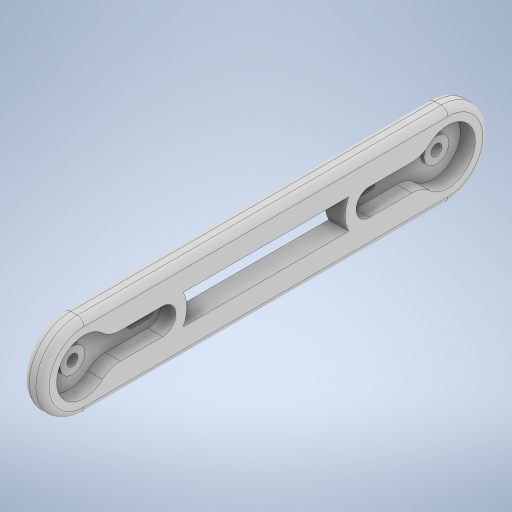
# Autodesk Inventor part: FemurHornSide
Saved by Autodesk Inventor 2024 (Build 280153000, 153)
## iProperties
Created: 2026-01-07
Part Number: FemurHornSide
Material: Generic
Document SubType Name: Modeling
Designer: Liam
Density: 1 g/cm^3
Appearance: Default
Mass: 22.8952 g
Surface Area: 100.934 cm^2
Volume: 22.8952 cm^3
Author: Liam
Autodesk Inventor part; units mm, degrees
ref_plane "YZ Plane" through (0, 0, 0) normal (1, 0, 0) x (0, 1, 0)
ref_plane "XZ Plane" through (0, 0, 0) normal (0, 1, 0) x (-1, 0, 0)
ref_plane "XY Plane" through (0, 0, 0) normal (0, 0, 1) x (1, 0, 0)
sketch "Sketch1" plane through (0, 0, 0) normal (1, 0, 0) x (0, 1, 0)
  line L0 (12.5, 55) -> (-12.5, 55)
  line L1 (-12.5, 55) -> (-12.5, -55)
  line L2 (-12.5, -55) -> (12.5, -55)
  line L3 (12.5, -55) -> (12.5, 55)
  arc A0 (12.5, 55) -> (-12.5, 55) centre (0, 55) ccw
  arc A1 (-12.5, -55) -> (12.5, -55) centre (0, -55) ccw
  circle A2 centre (0, 55) radius 1.65
  circle A3 centre (0, 55) radius 3.75
  circle A4 centre (0, 55) radius 8.25
  line L4 (4, 55) -> (-4, 55)
  line L5 (-4, 55) -> (-4, 27.25)
  line L6 (-4, 27.25) -> (4, 27.25)
  line L7 (4, 27.25) -> (4, 55)
  circle A5 centre (0, 31) radius 1.65
  circle A6 centre (0, 36) radius 1.65
  line L8 (1.65, 36) -> (1.65, 31)
  line L9 (-1.65, 36) -> (-1.65, 31)
  line L10 (12.5, 0) -> (-12.5, 0) construction
  circle A7 centre (0, -55) radius 1.65
  circle A8 centre (0, -55) radius 3.75
  circle A9 centre (0, -55) radius 8.25
  line L11 (-4, -55) -> (-4, -27.25)
  line L12 (-4, -27.25) -> (4, -27.25)
  line L13 (4, -27.25) -> (4, -55)
  circle A10 centre (0, -31) radius 1.65
  circle A11 centre (0, -36) radius 1.65
  line L14 (1.65, -36) -> (1.65, -31)
  line L15 (-1.65, -36) -> (-1.65, -31)
  line L16 (4.5, 25) -> (-4.5, 25)
  line L17 (-4.5, 25) -> (-4.5, -25)
  line L18 (-4.5, -25) -> (4.5, -25)
  line L19 (4.5, -25) -> (4.5, 25)
  line L20 (4.5, 25) -> (-4.5, -25) construction
  line L21 (-4.5, 25) -> (4.5, -25) construction
  arc A12 (-4.5, 25) -> (4.5, 25) centre (0, 33.9303) ccw
  arc A13 (4.5, -25) -> (-4.5, -25) centre (0, -33.9303) ccw
  point P0 (0, 0)
  point P1 (0, 55)
  point P2 (-4, -47.7846)
  point P3 (4, -47.7846)
  point P4 (4, 47.7846)
  point P5 (-4, 47.7846)
  point P6 (0, 0)
  point P7 (3.75, 55)
  point P8 (-3.75, 55)
  dimension "d0" = 110
  dimension "d1" = 55
  dimension "d2" = 12.5
  dimension "d3" = 25
  dimension "d4" = 3.3
  dimension "d5" = 7.5
  dimension "d6" = 16.5
  dimension "d7" = 8
  dimension "d8" = 4
  dimension "d10" = 36
  dimension "d11" = 3.3
  dimension "d12" = 24
  dimension "d13" = 4
  dimension "d14" = 3.3
  dimension "d15" = 5
  dimension "d16" = 4
  dimension "d34" = 50
  dimension "d35" = 8
  dimension "d36" = 8
  dimension "d37" = 10
  dimension "d38" = 10
  constraints: 44 end point, 16 point on circle, 14 centre point, 13 symmetric about line, 8 midpoint, 6 parallel, 5 coincident, 3 horizontal, 3 perpendicular, 2 tangent, 2 vertical, 1 point on line, 5 other
  measures "d0" distance between parallel lines of L2 L0
  measures "d1" distance from line of L2 point (0, 0)
  measures "d2" distance from line of L1 point (0, 0)
  measures "d3" distance of L1.end L2.end
  measures "d4" diameter of A2
  measures "d5" diameter of A3
  measures "d6" diameter of A4
  measures "d7" distance of L5.end L6.end
  measures "d8" distance from line of L5 A0.centre
  measures "d11" diameter of A5
  measures "d12" distance of A5.centre point (0, 55)
  measures "d13" distance from line of L5 A5.centre
  measures "d14" diameter of A6
  measures "d15" distance of A5.centre A6.centre
  measures "d16" distance from line of L5 A6.centre
  measures "d34" distance between parallel lines of L18 L16
  measures "d35" distance between parallel lines of L1 L17
  measures "d36" distance between parallel lines of L3 L19
  measures "d37" radius of A12
  measures "d38" radius of A13
extrude "Extrusion1" add sketch "Sketch1" along normal blind 4.5 contours L3 L2 A9 L13 L12 L11 L1 L0 A4 L5 L6 L7 | L0 A4 A0 | A1 L2 A9 | A12 L16 | L18 A13
extrude "Extrusion2" add sketch "Sketch1" against normal blind 1.5 contours L3 L2 A9 L13 L12 L11 L1 L0 A4 L5 L6 L7 | L0 A4 A0 | A4 L7 L0 | L0 A3 A4 | A1 L2 A9 | L7 A4 L5 L0 A3 | L0 L5 A4 | L7 L6 L5 A4 | A9 L2 A8 | L2 L13 A9 | A3 L0 A2 | L0 A2 A3 | L2 A8 L11 A9 L13 | A9 L11 L12 L13 | A9 L11 L2 | A8 L2 A7 | L2 A7 A8 | A12 L16 | L18 A13
extrude "Extrusion3" add sketch "Sketch1" along normal blind 1 contours A3 L0 A2 | L0 A2 A3 | A8 L2 A7 | L2 A7 A8
fillet "Fillet1" radius 4 4 edges at (2.25, -4, 27.25) (2.25, 4, 27.25) (2.25, -4, -27.25) (2.25, 4, -27.25)
fillet "Fillet2" radius 8 4 edges at (2.25, -4, -47.7846) (2.25, 4, -47.7846) (2.25, -4, 47.7846) (2.25, 4, 47.7846)
fillet "Fillet3" radius 2 8 edges at (4.5, 0, 67.5) (4.5, -12.5, 0) (4.5, 0, -67.5) (4.5, 12.5, 0) (-1.5, 0, -67.5) (-1.5, -12.5, 0) (-1.5, 0, 67.5) (-1.5, 12.5, 0)
equation "\"d0\" = FEMUR_X"
equation "\"d1\" = 0.5 * FEMUR_X"
equation "\"d2\" = 0.5 * FEMUR_WIDTH"
equation "\"d3\" = FEMUR_WIDTH"
equation "\"d4\" = HornScrewDiameter"
equation "\"d5\" = HornCentreDiameter"
equation "\"d6\" = HornDiameter"
equation "\"d7\" = HornWidth"
equation "\"d8\" = 0.5 * HornWidth"
equation "\"d10\" = HornLength"
equation "\"d11\" = HornScrewDiameter"
equation "\"d12\" = HornScrewX"
equation "\"d13\" = 0.5 * HornWidth"
equation "\"d14\" = HornScrewDiameter"
equation "\"d15\" = HornScrewLen"
equation "\"d16\" = 0.5 * HornWidth"
equation "\"d17\" = FEMUR_HEIGHT - HORN_HEIGHT"
equation "\"d19\" = HORN_HEIGHT"
equation "\"d21\" = HornCentreHeight"
equation "\"d23\" = 0.5 * HornWidth"
equation "\"d24\" = HornFillet"
equation "\"d25\" = PART_FILLET"
equation "\"FEMUR_X\" = 110"
equation "\"FEMUR_WIDTH\" = 25"
equation "\"HornScrewDiameter\" = 3.3"
equation "\"HornCentreDiameter\" = 7.5"
equation "\"HornDiameter\" = 16.5"
equation "\"HornWidth\" = 8"
equation "\"HornLength\" = 36"
equation "\"HornScrewLen\" = 5"
equation "\"FEMUR_HEIGHT\" = 6"
equation "\"HORN_HEIGHT\" = 1.5"
equation "\"HornCentreHeight\" = 1"
equation "\"HornFillet\" = 8"
equation "\"PART_FILLET\" = 2"
equation "\"HornScrewX\" = 24"
body "Solid1"
